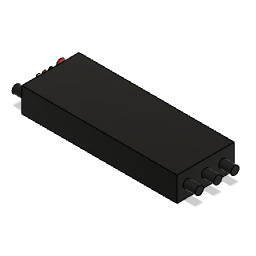
_20a brushless esc.c34dac7c-07c5-48fb-a4a8-653e6f9bd770 (Autodesk Fusion 360 design; units mm, degrees)
Autodesk Fusion 360 part; units mm, degrees
sketch "Sketch1" plane through (0, 0, 0) normal (0, 1, 0) x (1, 0, 0)
  line L0 (0, 0) -> (38, 0)
  line L1 (38, 0) -> (38, 14)
  line L2 (38, 14) -> (0, 14)
  line L3 (0, 14) -> (0, 0)
  line L4 (3.9603, 3.1256) -> (35.9564, 3.1256) construction
  line L5 (35.9564, 3.1256) -> (35.9564, 11.1256) construction
  line L6 (35.9564, 11.1256) -> (3.9603, 11.1256) construction
  line L7 (3.9603, 11.1256) -> (3.9603, 3.1256) construction
  dimension "d1" = 14
  dimension "d2" = 38
  constraint horizontal L0
  constraint vertical L1
  constraint horizontal L2
  constraint vertical L3
  constraint coincident L0.start L3.end
  constraint perpendicular L4 L5
  constraint parallel L4 L6
  constraint parallel L5 L7
  measures "d1" distance of L0.start L2.end
  measures "d2" distance of L0.start L0.end
extrude "Extrude1" add sketch "Sketch1" against normal blind 6
cylinder "CylinderPrimitive1" add diameter 2 height 3 placed x (0, 0, -1) y (0, 1, 0) z (1, 0, 0) at (38, -3, -2.4977)
sketch "Sketch3" plane through (38, 0, 0) normal (1, 0, 0) x (0, 0, -1)
  circle A0 centre (2.4977, -3) radius 1
  line L0 (14, 0) -> (0, 0)
  line L1 (0, 0) -> (0, -6)
  line L2 (0, -6) -> (14, -6)
  line L3 (14, -6) -> (14, 0)
cylinder "CylinderPrimitive2" add diameter 2 height 3 placed x (0, 0, -1) y (0, 1, 0) z (1, 0, 0) at (38, -3, -7)
cylinder "CylinderPrimitive3" add diameter 2 height 3 placed x (0, 0, -1) y (0, 1, 0) z (1, 0, 0) at (38, -3.0833, -11.2079)
sketch "Sketch5" plane through (0, 0, 0) normal (-1, 0, 0) x (0, 0, 1)
  line L0 (0, 0) -> (-14, 0)
  line L1 (-14, 0) -> (-14, -6)
  line L2 (-14, -6) -> (0, -6)
  line L3 (0, -6) -> (0, 0)
cylinder "CylinderPrimitive4" add diameter 2 height 3 placed x (0, 0, 1) y (0, 1, 0) z (-1, 0, 0) at (0, -3, -12.5)
cylinder "CylinderPrimitive5" add diameter 2 height 3 placed x (0, 0, 1) y (0, 1, 0) z (-1, 0, 0) at (0, -3, -1.6)
cylinder "CylinderPrimitive6" add diameter 1 height 3 placed x (0, 0, 1) y (0, 1, 0) z (-1, 0, 0) at (0, -3, -10)
cylinder "CylinderPrimitive7" add diameter 1 height 3 placed x (0, 0, 1) y (0, 1, 0) z (-1, 0, 0) at (0, -3, -8.5)
cylinder "CylinderPrimitive8" add diameter 1 height 3 placed x (0, 0, 1) y (0, 1, 0) z (-1, 0, 0) at (0, -3, -7)
named bodies: "ESC"
